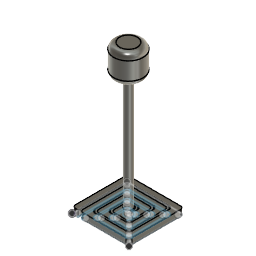
shifter_v2 (Autodesk Fusion 360 design; units mm, degrees)
Autodesk Fusion 360 part; units mm, degrees
note: some values were not read from the file. Set by a fixed rule: which sketch regions a step uses.
sketch "Sketch1" plane through (0, 0, 0) normal (0, 0, 1) x (1, 0, 0)
  line L0 (29, 1.5) -> (29, 26.5)
  line L1 (27.5, 28) -> (1.5, 28)
  line L2 (0, 26.5) -> (0, 1.5)
  line L3 (3, 0) -> (3, 23.5595)
  line L4 (4.5, 25.0595) -> (24.5, 25.0595)
  line L5 (26, 23.5595) -> (26, 4.5)
  line L6 (24.5, 3) -> (8.5, 3)
  line L7 (4, 3) -> (4, 1.5)
  line L8 (4, 3) -> (4, 22.4878)
  line L9 (5.5, 23.9878) -> (23.5, 23.9878)
  line L10 (25, 22.4878) -> (25, 5.5)
  line L11 (23.5, 4) -> (9.5, 4)
  line L12 (8, 5.5) -> (8, 18.4723)
  line L13 (9.5, 19.9723) -> (19.5, 19.9723)
  line L14 (21, 18.4723) -> (21, 9.5)
  line L15 (19.5, 8) -> (13.5173, 8)
  line L16 (12.0173, 9.5) -> (12.0173, 14.3549)
  line L17 (14.0173, 16.3549) -> (15.0961, 16.3549)
  line L18 (17.0961, 14.3549) -> (17.0961, 11)
  line L19 (7, 4.5) -> (7, 19.6029)
  line L20 (8.5, 21.1029) -> (20.5, 21.1029)
  line L21 (22, 19.6029) -> (22, 8.5)
  line L22 (20.5, 7) -> (12.5, 7)
  line L23 (11, 8.5) -> (11, 15.5643)
  line L24 (12.5, 17.0643) -> (16.5, 17.0643)
  line L25 (18, 15.5643) -> (18, 12.3765)
  line L26 (1.5, 0) -> (3, 0)
  line L27 (5.5, 0) -> (27.5, 0)
  circle A0 centre (14.675, 14.0515) radius 2
  arc A1 (1.5, 28) -> (0, 26.5) centre (1.5, 26.5) ccw
  arc A2 (0, 1.5) -> (1.5, 0) centre (1.5, 1.5) ccw
  arc A3 (4.5, 25.0595) -> (3, 23.5595) centre (4.5, 23.5595) ccw
  arc A4 (26, 23.5595) -> (24.5, 25.0595) centre (24.5, 23.5595) ccw
  arc A5 (29, 26.5) -> (27.5, 28) centre (27.5, 26.5) ccw
  arc A6 (27.5, 0) -> (29, 1.5) centre (27.5, 1.5) ccw
  arc A7 (4, 1.5) -> (5.5, 0) centre (5.5, 1.5) ccw
  arc A8 (5.5, 23.9878) -> (4, 22.4878) centre (5.5, 22.4878) ccw
  arc A9 (25, 22.4878) -> (23.5, 23.9878) centre (23.5, 22.4878) ccw
  arc A10 (23.5, 4) -> (25, 5.5) centre (23.5, 5.5) ccw
  arc A11 (24.5, 3) -> (26, 4.5) centre (24.5, 4.5) ccw
  arc A12 (7, 4.5) -> (8.5, 3) centre (8.5, 4.5) ccw
  arc A13 (8, 5.5) -> (9.5, 4) centre (9.5, 5.5) ccw
  arc A14 (9.5, 19.9723) -> (8, 18.4723) centre (9.5, 18.4723) ccw
  arc A15 (8.5, 21.1029) -> (7, 19.6029) centre (8.5, 19.6029) ccw
  arc A16 (22, 19.6029) -> (20.5, 21.1029) centre (20.5, 19.6029) ccw
  arc A17 (21, 18.4723) -> (19.5, 19.9723) centre (19.5, 18.4723) ccw
  arc A18 (20.5, 7) -> (22, 8.5) centre (20.5, 8.5) ccw
  arc A19 (19.5, 8) -> (21, 9.5) centre (19.5, 9.5) ccw
  arc A20 (11, 8.5) -> (12.5, 7) centre (12.5, 8.5) ccw
  arc A21 (12.5, 17.0643) -> (11, 15.5643) centre (12.5, 15.5643) ccw
  arc A22 (18, 15.5643) -> (16.5, 17.0643) centre (16.5, 15.5643) ccw
  arc A23 (17.0961, 11) -> (18, 12.3765) centre (16.5, 12.3765) ccw
  arc A24 (14.0173, 16.3549) -> (12.0173, 14.3549) centre (14.0173, 14.3549) ccw
  arc A25 (17.0961, 14.3549) -> (15.0961, 16.3549) centre (15.0961, 14.3549) ccw
  arc A26 (12.0173, 9.5) -> (13.5173, 8) centre (13.5173, 9.5) ccw
  point P0 (29, 0)
  point P1 (0, 28)
  dimension "d1" = 29
  dimension "d2" = 28
  dimension "d3" = 4
  dimension "d4" = 1.5
  dimension "d5" = 2
  dimension "d15" = 1.5
  constraint horizontal L26
  constraint vertical L0
  constraint horizontal L1
  constraint vertical L2
  constraint perpendicular L1 L3
  constraint perpendicular L0 L4
  constraint perpendicular L5 L26
  constraint perpendicular L5 L6
  constraint perpendicular L6 L7
  constraint perpendicular L6 L8
  constraint perpendicular L5 L9
  constraint perpendicular L9 L10
  constraint perpendicular L8 L11
  constraint perpendicular L9 L12
  constraint perpendicular L10 L13
  constraint perpendicular L9 L14
  constraint perpendicular L14 L15
  constraint perpendicular L15 L16
  constraint perpendicular L16 L17
  constraint perpendicular L15 L18
  constraint perpendicular L6 L19
  constraint perpendicular L19 L20
  constraint perpendicular L20 L21
  constraint perpendicular L21 L22
  constraint perpendicular L13 L23
  constraint perpendicular L23 L24
  constraint perpendicular L13 L25
  constraint collinear L26 L27
  constraint coincident P1 L1
  constraint coincident P1 L2
  constraint tangent L1 A1
  constraint tangent L2 A1
  constraint coincident origin L2
  constraint coincident origin L26
  constraint tangent L2 A2
  constraint tangent L26 A2
  constraint equal A1 A2
  constraint tangent L4 A3
  constraint tangent L3 A3
  constraint equal A1 A3
  constraint tangent L5 A4
  constraint tangent L4 A4
  constraint equal A1 A4
  constraint tangent L0 A5
  constraint tangent L1 A5
  constraint equal A1 A5
  constraint coincident P0 L0
  constraint coincident P0 L27
  constraint tangent L0 A6
  constraint tangent L27 A6
  constraint equal A1 A6
  constraint tangent L7 A7
  constraint tangent L27 A7
  constraint equal A1 A7
  constraint tangent L8 A8
  constraint tangent L9 A8
  constraint equal A1 A8
  constraint tangent L9 A9
  constraint tangent L10 A9
  constraint equal A1 A9
  constraint tangent L10 A10
  constraint tangent L11 A10
  constraint equal A1 A10
  constraint tangent L6 A11
  constraint tangent L5 A11
  constraint equal A1 A11
  constraint tangent L19 A12
  constraint tangent L6 A12
  constraint equal A1 A12
  constraint tangent L11 A13
  constraint tangent L12 A13
  constraint equal A1 A13
  constraint tangent L12 A14
  constraint tangent L13 A14
  constraint equal A1 A14
  constraint tangent L19 A15
  constraint tangent L20 A15
  constraint equal A1 A15
  constraint tangent L20 A16
  constraint tangent L21 A16
  constraint equal A1 A16
  constraint tangent L13 A17
  constraint tangent L14 A17
  constraint equal A1 A17
  constraint tangent L21 A18
  constraint tangent L22 A18
  constraint equal A1 A18
  constraint tangent L14 A19
  constraint tangent L15 A19
  constraint equal A1 A19
  constraint tangent L22 A20
  constraint tangent L23 A20
  constraint equal A1 A20
  constraint tangent L23 A21
  constraint tangent L24 A21
  constraint equal A1 A21
  constraint tangent L24 A22
  constraint tangent L25 A22
  constraint equal A1 A22
  constraint tangent L25 A23
  constraint equal A1 A23
  constraint coincident L18.end A23.start
  constraint tangent L16 A24
  constraint tangent L17 A24
  constraint tangent L17 A25
  constraint tangent L18 A25
  constraint equal A24 A25
  constraint tangent L15 A26
  constraint tangent L16 A26
  measures "d1" distance of origin P0
  measures "d2" distance of origin P1
  measures "d3" diameter of A0
  measures "d4" radius of A1
  measures "d5" radius of A24
  measures "d15" radius of A26
extrude "Extrude1" add sketch "Sketch1" along normal blind 3
extrude "Extrude2" add sketch "Sketch1" along normal blind 61 contours A0
sketch "Sketch2" plane through (0, 0, 61) normal (0, 0, 1) x (-1, 0, 0)
  circle A0 centre (-14.675, -14.0515) radius 2
  circle A1 centre (-14.675, -14.0515) radius 7.5
  dimension "d10" = 15
  constraint concentric A0 A1
  measures "d10" diameter of A1
extrude "Extrude3" add sketch "Sketch2" along normal blind 15 contours A0 | A1
fillet "Fillet1" radius 3 2 edges at (21.6674, 16.7636, 76) (21.6674, 16.7636, 61)
equation "d8 = 36 mm + 25 mm"
